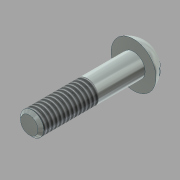
# Autodesk Inventor part: Round Head Machine Screw
Saved by Autodesk Inventor 2011 SP2 (Build 150309200, 309)
## iProperties
Created: 2014-10-09
Part Number: Round Head Machine Screw
Document SubType Name: Modeling
Designer: Greg Pavlik
Density: 1 g/cm^3
Author: Greg Pavlik
Autodesk Inventor part; units mm, degrees
ref_plane "YZ Plane" through (0, 0, 0) normal (1, 0, 0) x (0, 1, 0)
ref_plane "XZ Plane" through (0, 0, 0) normal (0, 1, 0) x (-1, 0, 0)
ref_plane "XY Plane" through (0, 0, 0) normal (0, 0, 1) x (1, 0, 0)
sketch "Sketch1" plane through (0, 0, 0) normal (0, 0, 1) x (1, 0, 0)
  line L0 (0, 0) -> (0, 21)
  arc A0 (3.873, 18) -> (0, 21) centre (0, 17) ccw
  line L1 (3.873, 18) -> (2, 18)
  line L2 (2, 18) -> (2, 0)
  line L3 (2, 0) -> (0, 0)
  dimension "Diameter" = 4
  dimension "Length" = 18
  dimension "d2" = 4
  dimension "d3" = 3
  constraints: 8 end point, 2 perpendicular, 2 point on circle, 1 centre point, 1 coincident, 1 parallel, 1 point on line, 1 vertical
  measures "Diameter" diameter of L2 L0
  measures "Length" distance between parallel lines of L3 L1
  measures "d2" radius of A0
  measures "d3" distance from line of L0.end L1
revolve "Revolution1" add sketch "Sketch1" angle 360 about axis through (0, 0, 0) along (0, 1, 0)
thread "Thread1" size "M4x0.7" class "6g" standard "ANSI Metric M Profile" length 10
sketch "Sketch2" plane through (0, 0, 0) normal (1, 0, 0) x (0, 1, 0)
  arc A0 (18, -3.873) -> (18, 3.873) centre (17, 0) ccw construction
  line L0 (0, 0) -> (21, 0) construction
  line L1 (21, 0.5) -> (19, 0.5)
  line L2 (19, 0.5) -> (19, -0.5)
  line L3 (19, -0.5) -> (21, -0.5)
  line L4 (21, -0.5) -> (21, 0.5)
  dimension "d7" = 2
  dimension "d8" = 1
  constraints: 10 end point, 2 horizontal, 2 parallel, 1 coincident, 1 perpendicular, 1 point on circle, 1 tangent, 1 other
  measures "d7" distance between parallel lines of L2 L4
  measures "d8" distance between parallel lines of L3 L1
extrude "Extrusion1" cut sketch "Sketch2" along normal through all both and the other way through all
chamfer "Chamfer1" distance 0.5 angle 45 1 edges at (-2, 0, 0)
equation "\"d2\" = Diameter"
equation "\"d3\" = 0.75 * Diameter"
equation "\"d7\" = 0.5 * Diameter"
equation "\"d8\" = 0.25 * Diameter"
body "Solid1"
